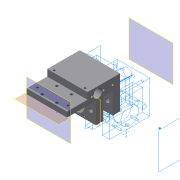
# Autodesk Inventor part: 01_Slide_camera_x_v0
Saved by Autodesk Inventor 2019.4 (Build 234330000, 330)
## iProperties
Created: 2020-10-27
Part Number: 01_Slide_camera_x_v0
Material: Generic
Document SubType Name: Modeling
Designer: diederichbenedict
Density: 1 g/cm^3
Appearance: Default
Author: diederichbenedict
Autodesk Inventor part; units mm, degrees
ref_plane "YZ Plane" through (0, 0, 0) normal (1, 0, 0) x (0, 1, 0)
ref_plane "XZ Plane" through (0, 0, 0) normal (0, 1, 0) x (-1, 0, 0)
ref_plane "XY Plane" through (0, 0, 0) normal (0, 0, 1) x (1, 0, 0)
ref_plane "Work Plane5" through (13.4046, 50.1721, 72.2727) normal (0, 1, 0) x (1, 0, 0)
sketch "Sketch7" plane through (13.4046, 50.1721, 72.2727) normal (0, 1, 0) x (1, 0, 0)
  circle A0 centre (6.5, 6.5) radius 2.5 construction
  circle A1 centre (48.5, 6.5) radius 2.5 construction
  line L0 (55, 2) -> (55, 11) construction
  line L1 (55, 35) -> (55, 44) construction
  circle A2 centre (48.5, 39.5) radius 2.5 construction
  circle A3 centre (6.5, 39.5) radius 2.5 construction
  line L2 (0, 35) -> (0, 44) construction
  line L3 (16.5, 85.8) -> (16.5, 84) construction
  line L4 (38.5, 85.8) -> (38.5, 84) construction
  line L5 (38.5, 84) -> (16.5, 84) construction
  line L6 (2, 0) -> (53, 0) construction
  line L7 (0, 13.3104) -> (55, 13.3104)
  line L8 (55, 13.3104) -> (55, 85.8)
  line L9 (55, 85.8) -> (0, 85.8)
  line L10 (0, 85.8) -> (0, 13.3104)
  point P0 (-13.4046, 72.2727)
  constraints: 22 end point, 5 vertical, 4 centre point, 3 horizontal, 2 parallel, 1 perpendicular, 1 point on line, 20 other
extrude "Extrusion7" add sketch "Sketch7" along normal blind 16
sketch "Sketch8" plane through (13.4046, 50.1721, -13.5273) normal (-1, 0, 0) x (0, 0, 1)
  circle A0 centre (50.2042, 7.5) radius 2.3
  circle A1 centre (30.4132, 7.5) radius 6
  point P0 (13.5273, -50.1721)
  dimension "d77" = 12
  constraints: 2 centre point, 2 other
  measures "d77" diameter of A1
extrude "Extrusion8" cut sketch "Sketch8" against normal through all contours A1
sketch "Sketch9" plane through (13.4046, 50.1721, 72.2727) normal (0, -1, 0) x (1, 0, 0)
  circle A0 centre (48.5, -44.5) radius 2.5
  circle A1 centre (6.5, -44.5) radius 2.5
  ellipse E0 centre (6.4724, -21.5) end of major axis (6.4724, -19) minor radius 2.5
  ellipse E1 centre (48.4722, -21.5) end of major axis (48.4722, -19) minor radius 2.5
  point P0 (-13.4046, -72.2727)
  point P1 (6.5, -6.5)
  point P2 (48.5, -6.5)
  constraints: 2 centre point, 12 other
hole "Hole1" at (19.9046, 50.1721, 65.7727) at (61.9046, 50.1721, 65.7727) at (61.9046, 50.1721, 27.7727) at (19.9046, 50.1721, 27.7727) at (61.8768, 50.1721, 50.7727) at (19.877, 50.1721, 50.7727) direction (0, 1, 0) diameter 2.9 end through all
sketch "Sketch10" plane through (68.4046, 50.1721, -13.5273) normal (0, 0, -1) x (-1, 0, 0)
  circle A0 centre (39, -26) radius 1
  circle A1 centre (16, -26) radius 1
  circle A2 centre (16, -3) radius 1
  circle A3 centre (39, -3) radius 1.1
  circle A4 centre (27.5, -14.5) radius 12
  circle A5 centre (27.5, -14.5) radius 10.8
  line L0 (55, 0) -> (0, 0) projected
  line L1 (11.5, -29) -> (43.5, -29)
  line L2 (43.5, -29) -> (43.5, 0)
  line L3 (43.5, 0) -> (11.5, 0)
  line L4 (11.5, 0) -> (11.5, -29)
  line L5 (11.5, -29) -> (43.5, 0) construction
  line L6 (43.5, -29) -> (11.5, 0) construction
  line L7 (0, 0) -> (11.5, 0)
  line L8 (43.5, 0) -> (55, 0)
  line L9 (55, 0) -> (43.5, 0)
  line L10 (43.5, 0) -> (43.5, -29)
  line L11 (43.5, -29) -> (55, -29)
  line L12 (55, -29) -> (55, 0)
  line L13 (11.5, -29) -> (0, -29)
  line L14 (0, -29) -> (0, 0)
  line L15 (0, 0) -> (11.5, 0)
  line L16 (11.5, 0) -> (11.5, -29)
  circle A6 centre (47.5, -14.5) radius 3 construction
  circle A7 centre (7.5, -14.5) radius 3 construction
  circle A8 centre (47.5, -14.5) radius 3.1
  circle A9 centre (7.5, -14.5) radius 3.1
  point P0 (68.4046, -50.1721)
  dimension "d50" = 24
  dimension "d51" = 32
  dimension "d67" = 6.2
  dimension "d68" = 6.2
  constraints: 32 end point, 10 centre point, 6 parallel, 3 horizontal, 3 perpendicular, 2 coincident, 2 collinear, 2 midpoint, 1 point on line, 14 other
  measures "d50" diameter of A4
  measures "d51" distance of L3.end L2.end
  measures "d67" diameter of A8
  measures "d68" diameter of A9
extrude "Extrusion9" add sketch "Sketch10" against normal blind 10 contours L12 L11 L2 L0 | L2 L1 L4 L0 | L4 L13 L14 L0
sketch "Sketch11" plane through (13.4046, 50.1721, 58.9623) normal (-1, 0, 0) x (0, 0, 1)
  line L0 (-62.4896, 0) -> (0, 0) projected
  line L1 (0, 16) -> (-72.4896, 16) projected
  circle A0 centre (-62.6569, 7.5) radius 1.625
  circle A1 centre (-46.6569, 7.5) radius 1.625
  point P0 (-58.9623, -50.1721)
  point P1 (-26.8659, 7.5)
  point P2 (-42.8659, 7.5)
  point P3 (-42.3508, 7.5759)
  constraints: 2 centre point, 6 other
hole "Hole2" at (13.4046, 57.6721, 12.3055) at (13.4046, 57.6721, -3.6945) direction (1, 0, 0) diameter 2.9 end through all
ref_plane "Work Plane6" through (68.4046, 66.1721, -83.5273) normal (0, 0, -1) x (-1, 0, 0)
ref_plane "Work Plane7" through (68.4046, 66.1721, 56.4727) normal (0, 0, -1) x (-1, 0, 0)
sketch "Sketch15" plane through (68.4046, 50.1721, 58.9623) normal (1, 0, 0) x (0, 0, -1)
  line L0 (0, 0) -> (62.4896, 0) projected
  line L1 (62.4896, -29) -> (62.4896, 0) projected
  line L2 (72.4896, -29) -> (62.4896, -29) projected
  line L3 (72.4896, -29) -> (72.4896, 16) projected
  line L4 (0, 16) -> (72.4896, 16) projected
  line L5 (0, 0) -> (0, 16) projected
  line L6 (72.4896, 16) -> (0, 16) projected
  line L7 (28, 16) -> (0, 16)
  line L8 (0, 16) -> (0, 7)
  line L9 (0, 7) -> (28, 7)
  line L10 (28, 7) -> (28, 16)
  point P0 (58.9623, -50.1721)
  dimension "d73" = 7
  dimension "d74" = 28
  constraints: 8 end point, 2 parallel, 2 point on line, 1 horizontal, 1 perpendicular
  measures "d73" distance between parallel lines of L9 L0
  measures "d74" distance between parallel lines of L5 L10
extrude "Extrusion12" cut sketch "Sketch15" against normal through all contours L5 L4 L10 L9
sketch "Sketch16" plane through (68.4046, 50.1721, 58.9623) normal (1, 0, 0) x (0, 0, -1)
  circle A0 centre (50.0764, 7.5) radius 1.625
  circle A1 centre (34.0764, 7.5) radius 1.625
  point P0 (58.9623, -50.1721)
  constraints: 2 centre point, 4 other
hole "Hole3" at (68.4046, 57.6721, 24.8859) at (68.4046, 57.6721, 8.8859) direction (-1, 0, 0) diameter 2.9 end through all
sketch "Sketch17" plane through (13.4046, 50.1721, 72.2727) normal (0, -1, 0) x (1, 0, 0)
  circle A0 centre (37.7, -36.8104) radius 1.25
  circle A1 centre (17.7, -36.8104) radius 1.25
  circle A2 centre (17.7, -16.8104) radius 1.25
  circle A3 centre (37.7, -16.8104) radius 1.25
  point P0 (-13.4046, -72.2727)
  constraints: 4 centre point, 8 other
hole "Hole4" at (51.1046, 50.1721, 35.4623) at (31.1046, 50.1721, 35.4623) at (51.1046, 50.1721, 55.4623) at (31.1046, 50.1721, 55.4623) direction (0, 1, 0) diameter 3.5 end through all counterbore diameter 7 counterbore depth 4
ref_plane "Work Plane8" through (68.4046, 50.1721, 16.4727) normal (0, 0, 1) x (1, 0, 0)
sketch "Sketch18" plane through (68.4046, 50.1721, 16.4727) normal (0, 0, 1) x (1, 0, 0)
  circle A0 centre (-27.5, -14.5) radius 12 projected
  circle A1 centre (-39, -3) radius 1.1 projected
  circle A2 centre (-16, -3) radius 1 projected
  circle A3 centre (-16, -26) radius 1 projected
  circle A4 centre (-39, -26) radius 1 projected
  circle A5 centre (-47.5, -14.5) radius 3.1 projected
  circle A6 centre (-7.5, -14.5) radius 3.1 projected
  line L0 (-55, -29) -> (0, -29) projected
  line L1 (0, -29) -> (0, 0) projected
  line L2 (-55, 0) -> (0, 0) projected
  line L3 (-55, 0) -> (-55, -29) projected
  point P0 (-68.4046, -50.1721)
extrude "Extrusion13" add sketch "Sketch18" along normal blind 3 and the other way blind 7
sketch "Sketch19" plane through (13.4046, 21.1721, -13.5273) normal (0, -1, 0) x (1, 0, 0)
  line L0 (55, 0) -> (0, 0) projected
  line L1 (55, 0) -> (55, 10) projected
  line L2 (0, 10) -> (55, 10) projected
  line L3 (0, 0) -> (0, 10) projected
  line L4 (55, 23) -> (55, 33) projected
  line L5 (0, 33) -> (55, 33) projected
  line L6 (0, 33) -> (0, 23) projected
  line L7 (55, 23) -> (0, 23) projected
  circle A0 centre (27.5, 4) radius 1.45
  circle A1 centre (27.5, 29) radius 1.45
  point P0 (-13.4046, 13.5273)
  dimension "d97" = 2.9
  dimension "d98" = 2.9
  dimension "d99" = 4
  dimension "d100" = 25
  constraints: 2 centre point
  measures "d97" diameter of A0
  measures "d98" diameter of A1
  measures "d99" distance from line of L0 A0.centre
  measures "d100" distance of A1.centre A0.centre
extrude "Extrusion14" cut sketch "Sketch19" against normal blind 6 contours A0 | A1
sketch "Sketch20" plane through (68.4046, 66.1721, -13.5273) normal (0, 0, -1) x (-1, 0, 0)
  line L0 (25.0893, -54) -> (21.9984, -53.9999) construction
  line L1 (32.966, -54.0001) -> (25.8869, -54) construction
  line L2 (21.9985, -45.9999) -> (32.9661, -46.0001) construction
  line L3 (33.4646, -49.8702) -> (33.4645, -53.5016) construction
  line L4 (21.4999, -53.5014) -> (21.4999, -49.87) construction
  line L5 (33.4645, -54.0001) -> (21.5, -54.0001) construction
  line L6 (21.5, -54.0001) -> (21.5, -45.9999) construction
  line L7 (21.5, -45.9999) -> (33.4645, -45.9999) construction
  line L8 (33.4645, -45.9999) -> (33.4645, -54.0001) construction
  line L9 (33.9645, -54.5001) -> (21, -54.5001)
  line L10 (21, -54.5001) -> (21, -45.4999)
  line L11 (21, -45.4999) -> (33.9645, -45.4999)
  line L12 (33.9645, -45.4999) -> (33.9645, -54.5001)
  circle A0 centre (7.5, -30.5) radius 3.1 projected
  circle A1 centre (47.5, -30.5) radius 3.1 projected
  circle A2 centre (39, -42) radius 1 projected
  circle A3 centre (16, -42) radius 1 projected
  circle A4 centre (16, -19) radius 1 projected
  circle A5 centre (39, -19) radius 1.1 projected
  circle A6 centre (27.5, -30.5) radius 12 projected
  line L13 (55, -45) -> (55, 0) projected
  line L14 (0, 0) -> (55, 0) projected
  line L15 (0, -45) -> (0, 0) projected
  line L16 (0, -45) -> (55, -45) projected
  line L17 (55, -45) -> (0, -45) projected
  line L18 (55, -45) -> (0, -45)
  line L19 (0, -45) -> (0, -59)
  line L20 (0, -59) -> (55, -59)
  line L21 (55, -59) -> (55, -45)
  point P0 (68.4046, -66.1721)
  point P1 (22.9955, -48.7255)
  dimension "d103" = 0.5
  dimension "d104" = 14
  constraints: 34 end point, 6 parallel, 3 perpendicular, 2 horizontal, 19 other
  measures "d103" distance between parallel lines of L8 L12
  measures "d104" distance of L19.end L18.end
extrude "Extrusion15" add sketch "Sketch20" against normal up to surface (10 mm away) contours L21 L20 L19 L16
sketch "Sketch22" plane through (68.4046, 50.1721, 9.4727) normal (0, 0, -1) x (-1, 0, 0)
  line L0 (21, -29.4999) -> (33.9645, -29.4999) projected
  line L1 (33.9645, -29.4999) -> (33.9645, -38.5001) projected
  line L2 (33.9645, -38.5001) -> (21, -38.5001) projected
  line L3 (21, -38.5001) -> (21, -29.4999) projected
  line L4 (21, -29.4999) -> (33.9645, -29.4999) projected
  circle A0 centre (7.5, -14.5) radius 3.1 projected
  circle A1 centre (47.5, -14.5) radius 3.1 projected
  circle A2 centre (39, -26) radius 1 projected
  circle A3 centre (16, -26) radius 1 projected
  circle A4 centre (16, -3) radius 1 projected
  circle A5 centre (39, -3) radius 1.1 projected
  circle A6 centre (27.5, -14.5) radius 12 projected
  line L5 (55, -43) -> (55, 16) projected
  line L6 (0, 16) -> (55, 16) projected
  line L7 (0, -43) -> (0, 16) projected
  line L8 (0, -43) -> (55, -43) projected
  line L9 (55, -43) -> (0, -43)
  line L10 (0, -43) -> (0, -28.9948)
  line L11 (0, -28.9948) -> (55, -28.9948)
  line L12 (55, -28.9948) -> (55, -43)
  point P0 (68.4046, -50.1721)
  constraints: 8 end point, 2 parallel, 1 horizontal, 1 perpendicular, 1 point on line
extrude "Extrusion17" add sketch "Sketch22" against normal up to surface (10 mm away) contours L8 L7 L11 L5
sketch "Sketch21" plane through (13.4046, 7.1721, -13.5273) normal (0, -1, 0) x (1, 0, 0)
  circle A0 centre (27.5, 4) radius 1.45 projected
  circle A1 centre (27.5, 29) radius 1.45 projected
  point P0 (-13.4046, 13.5273)
extrude "Extrusion16" cut sketch "Sketch21" against normal up to surface round surface about axis through (40.9046, 35.6721, -13.5273) along (0, 0, 1) radius 12 far side no
body "Solid2"
